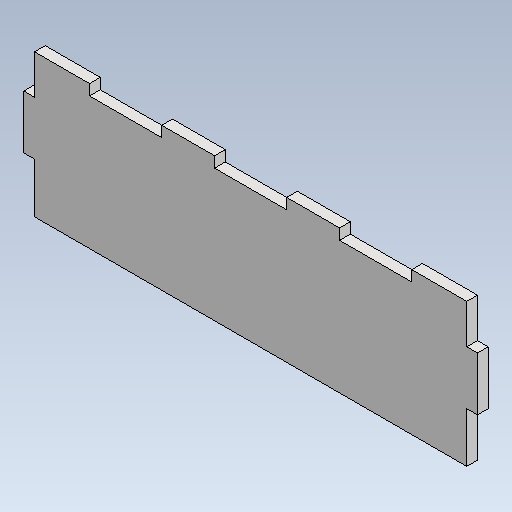
# Autodesk Inventor part: bed_acrylic_upper_floort
Saved by Autodesk Inventor 2025 (Build 290162000, 162)
## iProperties
Created: 2025-08-24
Part Number: bed_acrylic_upper_floort
Material: Generic
Document SubType Name: Modeling
Designer: HP
Density: 1 g/cm^3
Appearance: Default
Author: HP
Autodesk Inventor part; units mm, degrees
ref_plane "YZ Plane" through (0, 0, 0) normal (1, 0, 0) x (0, 1, 0)
ref_plane "XZ Plane" through (0, 0, 0) normal (0, 1, 0) x (-1, 0, 0)
ref_plane "XY Plane" through (0, 0, 0) normal (0, 0, 1) x (1, 0, 0)
sketch "Sketch1" plane through (0, 0, 0) normal (0, 0, 1) x (1, 0, 0)
  line L0 (-63.5, -20) -> (63.5, -20)
  line L1 (63.5, -20) -> (63.5, 20)
  line L2 (63.5, 20) -> (-63.5, 20)
  line L3 (-63.5, 20) -> (-63.5, -20)
  line L4 (-63.5, -20) -> (63.5, 20) construction
  line L5 (63.5, -20) -> (-63.5, 20) construction
  line L6 (-63.5, 9) -> (-60.5, 9)
  line L7 (-60.5, 9) -> (-60.5, -6) construction
  line L8 (-60.5, -6) -> (-63.5, -6)
  line L9 (-63.5, -6) -> (-63.5, 9)
  line L10 (-63.5, 9) -> (-60.5, -6) construction
  line L11 (-60.5, 9) -> (-63.5, -6) construction
  line L12 (-45.1, 20) -> (-24.9, 20)
  line L13 (-24.9, 20) -> (-24.9, 17)
  line L14 (-24.9, 17) -> (-45.1, 17)
  line L15 (-45.1, 17) -> (-45.1, 20)
  line L16 (-45.1, 20) -> (-24.9, 17) construction
  line L17 (-24.9, 20) -> (-45.1, 17) construction
  line L18 (-10.1, 20) -> (10.1, 20)
  line L19 (10.1, 20) -> (10.1, 17)
  line L20 (10.1, 17) -> (-10.1, 17)
  line L21 (-10.1, 17) -> (-10.1, 20)
  line L22 (-10.1, 20) -> (10.1, 17) construction
  line L23 (10.1, 20) -> (-10.1, 17) construction
  line L24 (24.9, 20) -> (45.1, 20)
  line L25 (45.1, 20) -> (45.1, 17)
  line L26 (45.1, 17) -> (24.9, 17)
  line L27 (24.9, 17) -> (24.9, 20)
  line L28 (24.9, 20) -> (45.1, 17) construction
  line L29 (45.1, 20) -> (24.9, 17) construction
  line L30 (-60.5, 9) -> (-60.5, 20)
  line L31 (-60.5, -6) -> (-60.5, -20)
  point P0 (0, 0)
  point P1 (-62, 1.5)
  point P2 (-63.5, 0)
  point P3 (-35, 18.5)
  point P4 (0, 18.5)
  point P5 (35, 18.5)
  point P6 (0, 20)
  point P7 (45.1, 20)
  point P8 (24.9, 20)
  point P9 (10.1, 20)
  point P10 (-45.1, 20)
  dimension "d0" = 127
  dimension "d1" = 40
  dimension "d2" = 3
  dimension "d3" = 15
  dimension "d4" = 20.2
  dimension "d5" = 3
  dimension "d6" = 20.2
  dimension "d7" = 3
  dimension "d8" = 20.2
  dimension "d9" = 3
  dimension "d10" = 35
  dimension "d11" = 35
  dimension "d16" = 1.5
  constraints: 64 end point, 12 midpoint, 10 parallel, 7 perpendicular, 5 horizontal, 4 collinear, 2 point on line, 1 vertical alignment
  measures "d0" distance between parallel lines of L1 L3
  measures "d1" distance between parallel lines of L0 L2
  measures "d2" distance between parallel lines of L7 L9
  measures "d3" distance between parallel lines of L8 L6
  measures "d4" distance of L13.end L14.end
  measures "d5" distance of L12.end L13.end
  measures "d6" distance of L19.end L21.start
  measures "d7" distance of L19.start L19.end
  measures "d8" distance of L25.end L27.start
  measures "d9" distance of L25.start L25.end
  measures "d10" distance of point (0, 18.5) point (-35, 18.5)
  measures "d11" distance of point (35, 18.5) point (0, 18.5)
  measures "d16" horizontal distance of point (-63.5, 0) point (-62, 1.5)
extrude "Extrusion1" add sketch "Sketch1" along normal blind 3 contours L3 L8 L31 L0 | L31 L8 L3 L6 L30 L2 L15 L14 L13 L21 L20 L19 L27 L26 L25 L1 L0 | L3 L2 L30 L6
extrude "Extrusion2" cut sketch "Sketch1" along normal through all contours L3 L8 L31 L0 | L3 L2 L30 L6 | L25 L26 L27 L2 | L2 L13 L14 L15 | L19 L20 L21 L2
mirror "Mirror1" about plane through (0, 0, 0) normal (1, 0, 0) of "Extrusion2"
equation "\"d5\" = d2"
equation "\"d6\" = d4"
equation "\"d7\" = d5"
equation "\"d8\" = d6"
equation "\"d9\" = d7"
equation "\"d11\" = d10"
body "Solid1"
